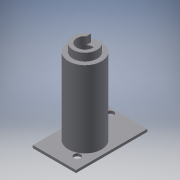
# Autodesk Inventor part: TORRE0.2
Saved by Autodesk Inventor 2016 (Build 200138000, 138)
## iProperties
Created: 2015-06-10
Part Number: TORRE0.2
Material: Generic
Document SubType Name: Modeling
Designer: pc
Density: 1 g/cm^3
Appearance: Default
Author: pc
Autodesk Inventor part; units mm, degrees
ref_plane "YZ Plane" through (0, 0, 0) normal (1, 0, 0) x (0, 1, 0)
ref_plane "XZ Plane" through (0, 0, 0) normal (0, 1, 0) x (-1, 0, 0)
ref_plane "XY Plane" through (0, 0, 0) normal (0, 0, 1) x (1, 0, 0)
sketch "Sketch1" plane through (0, 0, 0) normal (0, 0, 1) x (1, 0, 0)
  line L0 (-17, 28) -> (0, 28)
  line L1 (0, 28) -> (0, 0)
  line L2 (0, 0) -> (-17, 0)
  line L3 (-17, 0) -> (-17, 28)
  dimension "d0" = 17
  dimension "d1" = 28
  constraints: 8 end point, 3 perpendicular, 1 coincident, 1 horizontal
  measures "d0" distance of L0.start L0.end
  measures "d1" distance of L0.end L1.end
extrude "Extrusion1" add sketch "Sketch1" along normal blind 1
sketch "Sketch2" plane through (0, 0, 1) normal (0, 0, 1) x (1, 0, 0)
  line L0 (-17, 28) -> (-17, 0) projected
  line L1 (0, 28) -> (-17, 28) projected
  line L2 (0, 0) -> (0, 28) projected
  line L3 (-17, 0) -> (0, 0) projected
  circle A0 centre (-12.5, 26) radius 1.35
  circle A1 centre (-4.5, 5) radius 1.35
  dimension "d4" = 2.7
  dimension "d5" = 2.7
  dimension "d6" = 4.5
  dimension "d7" = 4.5
  dimension "d8" = 2
  dimension "d9" = 5
  constraints: 2 centre point
  measures "d4" diameter of A0
  measures "d5" diameter of A1
  measures "d6" distance from line of A0.centre L0
  measures "d7" distance from line of A1.centre L2
  measures "d8" distance from line of L1 A0.centre
  measures "d9" distance from line of A1.centre L3
extrude "Extrusion2" cut sketch "Sketch2" against normal through all contours A0 | A1
sketch "Sketch3" plane through (0, 0, 1) normal (0, 0, 1) x (1, 0, 0)
  circle A0 centre (-12.5, 26) radius 1.35 projected
  circle A1 centre (-4.5, 5) radius 1.35 projected
  line L0 (0, 28) -> (-17, 28) projected
  line L1 (-17, 28) -> (-17, 0) projected
  line L2 (-17, 0) -> (0, 0) projected
  line L3 (0, 0) -> (0, 28) projected
  circle A2 centre (-8.5, 12.047) radius 6.5
  dimension "d12" = 13
  dimension "d13" = 12.047
  constraints: 1 centre point
  measures "d12" diameter of A2
  measures "d13" distance from line of L2 A2.centre
extrude "Extrusion3" add sketch "Sketch3" along normal blind 30 contours A2
sketch "Sketch4" plane through (-8.5, 12.047, 31) normal (0, 0, 1) x (1, 0, 0)
  circle A0 centre (0, 0) radius 6.5 projected
  circle A1 centre (0, 0) radius 3.25
  point P0 (8.5, -12.047)
  dimension "d16" = 6.5
  constraints: 1 centre point, 1 coincident
  measures "d16" diameter of A1
sketch "Sketch5" plane through (0, 0, 0) normal (0, 0, -1) x (-1, 0, 0)
  circle A0 centre (8.5, 12.047) radius 6.5 projected
  circle A1 centre (8.5, 12.047) radius 5
  point P0 (0, 0)
  dimension "d17" = 10
  constraints: 1 centre point, 1 coincident
  measures "d17" diameter of A1
loft "Loft1" cut profiles "Sketch5", "Sketch4" contours A1 / A1
sketch "Sketch6" plane through (-8.5, 12.047, 31) normal (0, 0, 1) x (1, 0, 0)
  circle A0 centre (0, 0) radius 3.25 projected
  circle A1 centre (0, 0) radius 4.75
  point P0 (8.5, -12.047)
  dimension "d26" = 9.5
  constraints: 1 centre point, 1 coincident
  measures "d26" diameter of A1
extrude "Extrusion6" add sketch "Sketch6" along normal blind 3
sketch "Sketch7" plane through (-8.5, 12.047, 34) normal (0, 0, 1) x (1, 0, 0)
  circle A0 centre (0, 0) radius 3.25 projected
  circle A1 centre (0, 0) radius 4.75 projected
  line L0 (2, 0) -> (-2, 0)
  line L1 (-2, 0) -> (-2, 6)
  line L2 (-2, 6) -> (2, 6)
  line L3 (2, 6) -> (2, 0)
  point P0 (8.5, -12.047)
  dimension "d29" = 4
  dimension "d30" = 2
  constraints: 8 end point, 2 parallel, 1 horizontal, 1 midpoint, 1 perpendicular
  measures "d29" distance of L0.start L0.end
  measures "d30" distance from line of A0.centre L3
extrude "Extrusion7" cut sketch "Sketch7" against normal up to surface (3 mm away) contours L3 L0 L1 A0 | A0 L1 A1 L3 | A1 L1 L2 L3 picked at (0, 1.0833) picked at (0.3414, 4.2128)
body "Solid1"
